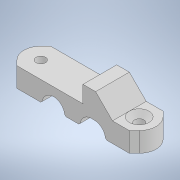
# Autodesk Inventor part: Magnet Mount Lower
Saved by Autodesk Inventor 2022 (Build 260153000, 153)
## iProperties
Created: 2022-04-23
Part Number: Magnet Mount Lower
Material: Generic
Document SubType Name: Modeling
Designer: Nick
Density: 1 g/cm^3
Appearance: Default
Author: Nick
Autodesk Inventor part; units mm, degrees
ref_plane "YZ Plane" through (0, 0, 0) normal (1, 0, 0) x (0, 1, 0)
sketch "Sketch1" plane through (0, 0, 0) normal (0, 0, 1) x (1, 0, 0)
  line L0 (0, 0) -> (28, 0)
  line L1 (28, 0) -> (28, 13)
  line L2 (28, 13) -> (0, 13)
  line L3 (0, 13) -> (0, 0)
  circle A0 centre (7, 0) radius 4
  circle A1 centre (21, 0) radius 4 construction
  line L4 (21, 0) -> (23, 0) construction
  line L5 (20.5, 0) -> (21.5, 0) construction
  line L6 (20.5, 4) -> (21.5, 4)
  line L7 (21.5, -4) -> (20.5, -4)
  arc A2 (20.5, 4) -> (20.5, -4) centre (20.5, 0) ccw
  arc A3 (21.5, -4) -> (21.5, 4) centre (21.5, 0) ccw
  point P0 (3, 0)
  point P1 (11, 0)
  point P2 (17, 0)
  point P3 (25, 0)
  point P4 (22, 0)
  point P5 (21, 0)
  point P6 (16.5, 0)
  point P7 (25.5, 0)
  dimension "d0" = 28
  dimension "d1" = 13
  dimension "d2" = 8
  dimension "d3" = 8
  dimension "d4" = 14
  dimension "d5" = 7
  dimension "d6" = 7
  dimension "d39" = 1
  dimension "d40" = 1
  constraints: 20 end point, 4 centre point, 4 point on circle, 4 tangent, 3 parallel, 3 point on line, 2 horizontal, 2 midpoint, 1 coincident, 1 equal radius, 1 perpendicular
  measures "d0" distance of L1.end L2.end
  measures "d1" distance of L0.end L1.end
  measures "d2" diameter of A0
  measures "d3" diameter of A1
  measures "d4" distance of L4.start A0.centre
  measures "d5" distance from line of L1 L4.start
  measures "d6" distance from line of A0.centre L3
  measures "d39" distance of L4.start point (22, 0)
  measures "d40" distance of L5.end L5.start
extrude "Extrusion1" add sketch "Sketch1" along normal blind 12 contours L3 L2 L1 L0 A3 L6 A2 A0
chamfer "Chamfer1" distance 6 angle 45 1 edges at (28, 13, 6)
sketch "Sketch2" plane through (0, 13, 12) normal (0, 1, 0) x (1, 0, 0)
  line L0 (0, 12) -> (0, 0) projected
  line L1 (0, 7.25) -> (11.5, 7.25)
  line L2 (11.5, 7.25) -> (11.5, 12)
  line L3 (22, 12) -> (0, 12) projected
  line L4 (17.5, 12) -> (17.5, 0)
  line L5 (11, 0) -> (3, 0) projected
  line L6 (0, 4.75) -> (11.5, 4.75)
  line L7 (11.5, 4.75) -> (11.5, 0)
  line L8 (11, 0) -> (3, 0) projected
  line L9 (11.5, 12) -> (17.5, 12)
  line L10 (17.5, 0) -> (11.5, 0)
  line L11 (0, 4.75) -> (0, 7.25)
  line L12 (11.5, 7.25) -> (11.5, 4.75)
  line L13 (0, 4.75) -> (11.5, 4.75)
  line L14 (11.5, 4.75) -> (11.5, 0)
  line L15 (11.5, 0) -> (0, 0)
  line L16 (0, 0) -> (0, 4.75)
  line L17 (11, 0) -> (16.5, 0) projected
  line L18 (11.5, 12) -> (14, 12)
  line L19 (14, 12) -> (14, 0)
  line L20 (14, 0) -> (11.5, 0)
  line L21 (11.5, 0) -> (11.5, 12)
  line L22 (0, 7.25) -> (0.5, 8)
  line L23 (0.5, 8) -> (1, 7.25)
  line L24 (2, 7.25) -> (2.5, 8)
  line L25 (2.5, 8) -> (3, 7.25)
  line L26 (4, 7.25) -> (4.5, 8)
  line L27 (4.5, 8) -> (5, 7.25)
  line L28 (6, 7.25) -> (6.5, 8)
  line L29 (6.5, 8) -> (7, 7.25)
  line L30 (8, 7.25) -> (8.5, 8)
  line L31 (8.5, 8) -> (9, 7.25)
  line L32 (0, 12) -> (0, 0) projected
  line L33 (0, 6) -> (11.5, 6) construction
  line L34 (0, 4.75) -> (0.5, 4)
  line L35 (0.5, 4) -> (1, 4.75)
  line L36 (2, 4.75) -> (2.5, 4)
  line L37 (2.5, 4) -> (3, 4.75)
  line L38 (4, 4.75) -> (4.5, 4)
  line L39 (4.5, 4) -> (5, 4.75)
  line L40 (6, 4.75) -> (6.5, 4)
  line L41 (6.5, 4) -> (7, 4.75)
  line L42 (8, 4.75) -> (8.5, 4)
  line L43 (8.5, 4) -> (9, 4.75)
  point P0 (17, 0)
  point P1 (3, 0)
  dimension "d12" = 6
  dimension "d13" = 2.5
  dimension "d14" = 11.5
  dimension "d41" = 2.5
  dimension "d42" = 0.75
  dimension "d43" = 1
  dimension "d46" = 2
  constraints: 76 end point, 14 symmetric about line, 8 point on line, 6 perpendicular, 5 horizontal, 4 parallel, 2 equal length, 2 midpoint, 1 collinear, 1 vertical, 20 other
  measures "d12" distance between parallel lines of L4 L2
  measures "d13" distance between parallel lines of L6 L1
  measures "d14" distance of L1.start L1.end
  measures "d41" distance of L19.end L20.end
  measures "d42" distance from line of L1 L22.end
  measures "d43" distance of L23.end L1.start
  measures "d46" distance of L1.start L24.start
extrude "Extrusion2" cut sketch "Sketch2" against normal blind 6
fillet "Fillet1" [suppressed]
chamfer "Chamfer2" distance 0.5 angle 45 4 edges at (3, 0, 6) (11, 0, 6) (16.5, 0, 6) (25.5, 0, 6)
ref_plane "Work Plane1" through (0, 0, 6) normal (0, 0, 1) x (1, 0, 0)
ref_plane "Work Plane3" through (14, 0, 12) normal (1, 0, 0) x (0, 0, -1)
sketch "Sketch5" plane through (28, 0, 0) normal (0, -1, 0) x (1, 0, 0)
  circle A0 centre (3.5, 6) radius 1.5
  line L0 (-28, 0) -> (-25.5, 0) projected
  line L1 (0, 0) -> (0, 12) projected
  circle A1 centre (3.5, 6) radius 3.5
  line L2 (0, 0) -> (0, 12) projected
  line L3 (-6, 12) -> (0, 12) projected
  line L4 (0, 12) -> (5.9853, 12)
  line L5 (0, 0) -> (-6, 0) projected
  line L6 (0, 0) -> (5.9853, 0)
  line L7 (5.9853, 0) -> (7.7426, 1.7574)
  line L8 (5.9853, 12) -> (7.7426, 10.2426)
  circle A2 centre (3.5, 6) radius 6
  line L9 (-28, 12) -> (-25.5, 12) projected
  line L10 (-28, 0) -> (-28, 12) projected
  line L11 (-25.5, 12) -> (-25.5, 0) projected
  line L12 (-16.5, 0) -> (-16.5, 12) projected
  line L13 (-16.5, 0) -> (-12, 0) projected
  line L14 (-16.5, 12) -> (-12, 12) projected
  line L15 (-2, 0) -> (0, 0) projected
  line L16 (-2, 12) -> (0, 12) projected
  line L17 (-12, 12) -> (-12, 0) projected
  line L18 (-2, 0) -> (-2, 12) projected
  point P0 (-2.5, 12)
  point P1 (-2.5, 0)
  point P2 (0, 6)
  dimension "d26" = 3
  dimension "d28" = 7
  dimension "d38" = 135
  constraints: 8 end point, 4 tangent, 3 centre point, 2 coincident, 2 equal length, 2 horizontal, 2 point on circle, 1 horizontal alignment, 1 midpoint
  measures "d26" diameter of A0
  measures "d28" diameter of A1
  measures "d38" angle of L6 L7
extrude "Extrusion3" add sketch "Sketch5" against normal blind 7 contours A0 | L1 A2 L6 | A1 | L1 A2 | A2 L7 L6 | L1 L4 A2 | L4 L8 A2
sketch "Sketch6" plane through (28, 7, 0) normal (0, 1, 0) x (1, 0, 0)
  arc A0 (7.7426, -10.2426) -> (7.7426, -1.7574) centre (3.5, -6) ccw projected
  point P0 (-28, 0)
hole "Hole1" at (31.5, 7, 6) direction (0, -1, 0) diameter 3.4 depth 8 clearance for "Flat Head Machine Screw" size "M3" standard "Ansi Metric M Profile"
mirror "Mirror2" about plane through (14, 0, 12) normal (1, 0, 0) of "Extrusion3", "Hole1"
chamfer "Chamfer3" distance 1.8 angle 45 1 edges at (31.5, 7, 4.3)
equation "\"d5\" = d6"
body "Solid1"
